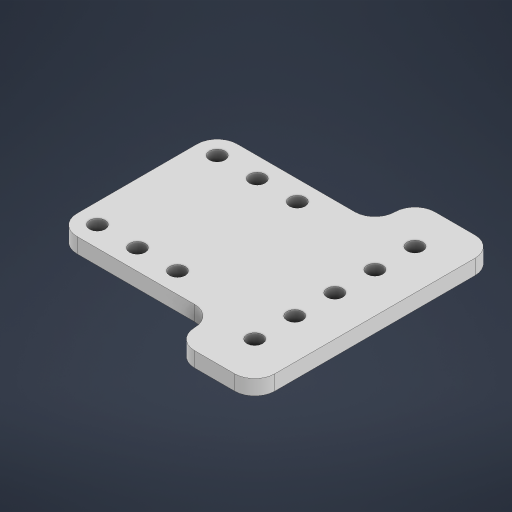
# Autodesk Inventor part: CLIM_009_BoBracket
Saved by Autodesk Inventor 2024.2 (Build 282272000, 272)
## iProperties
Created: 2024-08-08
Part Number: CLIM_009_BoBracket
Material: Generic
Document SubType Name: Modeling
Designer: Bryan
Density: 1 g/cm^3
Appearance: Default
Author: Bryan
Autodesk Inventor part; units mm, degrees
ref_plane "YZ Plane" through (0, 0, 0) normal (1, 0, 0) x (0, 1, 0)
ref_plane "XZ Plane" through (0, 0, 0) normal (0, 1, 0) x (-1, 0, 0)
ref_plane "XY Plane" through (0, 0, 0) normal (0, 0, 1) x (1, 0, 0)
sketch "Sketch1" plane through (0, 0, 0) normal (0, 1, 0) x (-1, 0, 0)
  circle A0 centre (0, 0) radius 2.4892
  line L0 (0, 0) -> (0, -25.4)
  circle A1 centre (0, -12.7) radius 2.4892
  circle A2 centre (0, -25.4) radius 2.4892
  circle A3 centre (0, -38.1) radius 2.4892
  circle A4 centre (0, -50.8) radius 2.4892
  circle A5 centre (56.3563, -6.45) radius 2.4892
  line L1 (56.3563, -6.45) -> (53.8671, -6.45) construction
  circle A6 centre (43.6563, -6.45) radius 2.4892
  circle A7 centre (30.9563, -6.45) radius 2.4892
  circle A8 centre (56.3563, -44.45) radius 2.4892
  circle A9 centre (43.6563, -44.45) radius 2.4892
  circle A10 centre (30.9562, -44.45) radius 2.4892
  line L2 (-12.7, 12.7) -> (12.7, 12.7)
  line L3 (12.7, 12.7) -> (12.7, -63.5)
  line L4 (12.7, -63.5) -> (-12.7, -63.5)
  line L5 (-12.7, -63.5) -> (-12.7, 12.7)
  line L6 (62.7062, 0) -> (12.7, 0)
  line L7 (12.7, 0) -> (12.7, -50.8)
  line L8 (12.7, -50.8) -> (62.7063, -50.8)
  line L9 (62.7063, -50.8) -> (62.7062, 0)
  point P0 (41.1671, -6.45)
  point P1 (28.4671, -6.45)
  point P2 (53.8671, -44.45)
  point P3 (41.1671, -44.45)
  point P4 (28.4671, -44.45)
  point P5 (12.7, -25.4)
  point P6 (12.7, 0)
  dimension "d9" = 4.9784
  dimension "d0" = 4.9784
  dimension "d1" = 25.4
  dimension "d4" = 12.7
  dimension "d12" = 12.7
  dimension "d15" = 38
  dimension "d18" = 25.4
  dimension "d19" = 76.2
  dimension "d20" = 12.7
  dimension "d21" = 12.7
  dimension "d22" = 18.2563
  dimension "d23" = 6.35
  dimension "d24" = 6.35
  dimension "d25" = 50.8
  constraints: 20 end point, 6 horizontal, 6 horizontal alignment, 6 vertical, 5 centre point, 4 parallel, 2 midpoint, 2 perpendicular, 1 coincident, 1 point on line, 30 other
  measures "d0" diameter of A0
  measures "d1" distance of L0.start L0.end
  measures "d4" distance of L0.start A1.centre
  measures "d12" distance of L1.start point (43.656, -6.45)
  measures "d15" distance of L1.start point (56.356, -44.45)
  measures "d18" distance of L3.end L4.end
  measures "d19" distance of L2.end L3.end
  measures "d20" distance from line of point (0, 0) L2
  measures "d21" distance of point (12.7, -25.4) A2.centre
  measures "d22" distance from line of L3 point (30.956, -44.45)
  measures "d23" distance from line of L8 point (56.356, -44.45)
  measures "d24" distance from line of L9 point (56.356, -44.45)
  measures "d25" distance of L8.end L6.start
extrude "Extrusion1" add sketch "Sketch1" along normal blind 4.7625
fillet "Fillet1" radius 6.35 8 edges at (-62.7062, 2.3813, 0) (-12.7, 2.3813, 0) (-12.7, 2.3813, 12.7) (12.7, 2.3813, 12.7) (-62.7063, 2.3813, -50.8) (-12.7, 2.3813, -50.8) (-12.7, 2.3813, -63.5) (12.7, 2.3813, -63.5)
body "Solid1"
